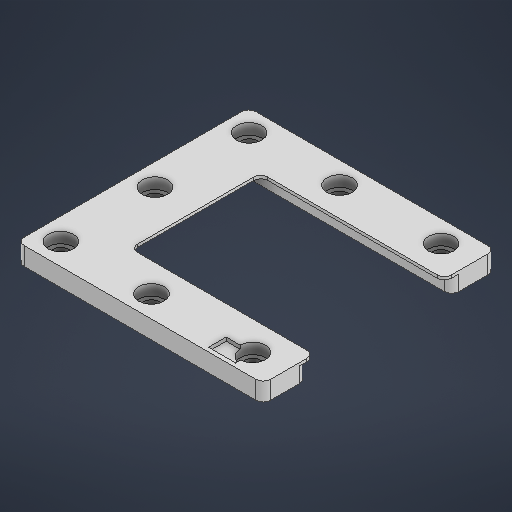
# Autodesk Inventor part: Flex Circuit Clamp V2
Saved by Autodesk Inventor 2027 (Build 310192060, 192F)
## iProperties
Created: 2026-05-04
Part Number: Flex Circuit Clamp V2
Material: Generic
Document SubType Name: Modeling
Designer: cfang
Density: 1 g/cm^3
Appearance: Default
Author: cfang
Autodesk Inventor part; units mm, degrees
ref_plane "YZ Plane" through (0, 0, 0) normal (1, 0, 0) x (0, 1, 0)
ref_plane "XZ Plane" through (0, 0, 0) normal (0, 1, 0) x (-1, 0, 0)
ref_plane "XY Plane" through (0, 0, 0) normal (0, 0, 1) x (1, 0, 0)
sketch "Sketch1" plane through (0, 0, 0) normal (0, 1, 0) x (-1, 0, 0)
  line L0 (-17, -16) -> (17, -16)
  line L1 (17, -16) -> (17, 16)
  line L2 (17, 16) -> (-17, 16)
  line L3 (-17, 16) -> (-17, -16)
  line L4 (-17, -16) -> (17, 16) construction
  line L5 (17, -16) -> (-17, 16) construction
  point P0 (0, 0)
  dimension "d0" = 32
  dimension "d1" = 34
  constraints: 12 end point, 2 midpoint, 2 parallel, 1 horizontal, 1 perpendicular
  measures "d0" distance of L0.end L1.end
  measures "d1" distance of L1.end L2.end
extrude "Extrusion1" add sketch "Sketch1" along normal blind 2.5
sketch "Sketch2" plane through (0, 2.5, 0) normal (0, 1, 0) x (1, 0, 0)
  line L0 (17, -16) -> (17, 16) projected
  line L1 (17, -10) -> (-10.85, -10)
  line L2 (-10.85, -10) -> (-10.85, 10)
  line L3 (-10.85, 10) -> (17, 10)
  line L4 (17, 10) -> (17, -10)
  point P0 (0, 0)
  point P1 (17, 10)
  dimension "d4" = 20
  dimension "d5" = 10
  dimension "d6" = 27.85
  constraints: 8 end point, 2 parallel, 1 horizontal, 1 perpendicular, 1 point on line
  measures "d4" distance of L1.end L2.end
  measures "d5" distance from line of L1 point (0, 0)
  measures "d6" distance of L1.start L1.end
extrude "Extrusion2" cut sketch "Sketch2" against normal through all
sketch "Sketch3" plane through (0, 2.5, 0) normal (0, 1, 0) x (1, 0, 0)
  line L0 (17, -10) -> (-10.85, -10) projected
  line L1 (-10.85, -10) -> (-10.85, 10) projected
  line L2 (-10.85, 10) -> (17, 10) projected
  line L3 (17, -10) -> (-10.85, -10)
  line L4 (-10.85, -10) -> (-10.85, -9)
  line L5 (-7.35, -9) -> (16, -9)
  line L6 (17, -10) -> (17, -10)
  line L7 (17, 10) -> (-10.85, 10)
  line L8 (-10.85, 10) -> (-10.85, 9)
  line L9 (-7.35, 9) -> (16, 9)
  line L10 (17, 10) -> (17, 10)
  line L11 (-10.85, -10) -> (-8.35, -10)
  line L12 (-8.35, -8) -> (-8.35, 8)
  line L13 (-8.35, 10) -> (-10.85, 10)
  line L14 (-10.85, 10) -> (-10.85, -10)
  arc A0 (17, -10) -> (16, -9) centre (16, -10) ccw
  arc A1 (-8.35, -8) -> (-7.35, -9) centre (-7.35, -8) ccw
  arc A2 (-7.35, 9) -> (-8.35, 8) centre (-7.35, 8) ccw
  arc A3 (16, 9) -> (17, 10) centre (16, 10) ccw
  point P0 (0, 0)
  point P1 (17, -9)
  point P2 (17, 9)
  point P3 (-7.5, -9)
  point P4 (-7.5, 9)
  point P5 (17, 10)
  dimension "d9" = 1
  dimension "d10" = 1
  dimension "d11" = 2.5
  dimension "d14" = 1
  constraints: 24 end point, 11 point on line, 8 point on circle, 8 tangent, 6 parallel, 4 centre point, 3 equal radius, 3 horizontal, 3 perpendicular
  measures "d9" distance between parallel lines of L0 L5
  measures "d10" distance between parallel lines of L2 L9
  measures "d11" distance between parallel lines of L1 L12
  measures "d14" radius of A0
extrude "Extrusion3" add sketch "Sketch3" against normal blind 0.4
sketch "Sketch4" plane through (0, 2.5, 0) normal (0, 1, 0) x (1, 0, 0)
  line L0 (-10.85, 10) -> (-10.85, -10) projected
  line L1 (-17, 16) -> (-17, -16) projected
  line L2 (-10.85, 10) -> (-10.85, -10) projected
  line L3 (-10.85, 10) -> (-10.85, -10) projected
  point P0 (0, 0)
  point P1 (12.55, -13)
  point P2 (-13.95, -13)
  point P3 (-13.95, 13)
  point P4 (12.55, 13)
  point P5 (-13.95, 0)
  point P6 (-1.45, -13)
  point P7 (-1.45, 13)
  dimension "d27" = 13
  dimension "d28" = 13
  dimension "d29" = 12.5
  dimension "d30" = 14
  dimension "d31" = 3.1
  constraints: 5 horizontal alignment, 4 vertical alignment
  measures "d27" distance of point (-13.95, -13) point (-13.95, 0)
  measures "d28" distance of point (-13.95, 0) point (-13.95, 13)
  measures "d29" distance of point (-1.45, -13) point (-13.95, -13)
  measures "d30" distance of point (12.55, -13) point (-1.45, -13)
  measures "d31" distance from line of point (-13.95, 0) L0
hole "Hole1" at (12.55, 2.5, 13) at (-13.95, 2.5, 13) at (-13.95, 2.5, -13) at (12.55, 2.5, -13) at (-1.45, 2.5, 13) at (-1.45, 2.5, -13) at (-13.95, 2.5, 0) direction (0, -1, 0) diameter 2.25 end through all counterbore diameter 3.5 counterbore depth 1.5
fillet "Fillet1" radius 1 6 edges at (-17, 1.25, 16) (-17, 1.25, -16) (17, 1.05, 10) (17, 1.25, 16) (17, 1.05, -10) (17, 1.25, -16)
sketch "Sketch5" plane through (0, 2.5, 0) normal (0, 1, 0) x (1, 0, 0)
  circle A0 centre (12.55, -13) radius 1.75 projected
  line L0 (12.6221, -15.435) -> (8.8746, -15.435)
  line L1 (8.8746, -15.435) -> (8.8746, -12.9967)
  line L2 (8.8746, -12.9967) -> (10.8, -12.9967)
  line L3 (12.6221, -15.435) -> (12.6221, -14.7485)
  point P0 (0, 0)
  constraints: 8 end point, 2 point on circle, 2 vertical, 1 horizontal, 1 parallel
extrude "Extrusion4" cut sketch "Sketch5" against normal blind 0.5 contours A0 L3 L0 L1 L2
equation "\"d5\" = 0.5 * d4"
equation "\"d10\" = d9"
equation "\"d28\" = d27"
body "Solid1"
